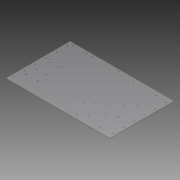
# Autodesk Inventor part: Mounting Board 1
Saved by Autodesk Inventor 2013 (Build 170138000, 138)
## iProperties
Created: 2013-01-21
Part Number: Mounting Board 1
Material: Polycarbonate, Clear
Document SubType Name: Modeling
Designer: Moses
Density: 1.2 g/cm^3
Mass: 570.089 g
Surface Area: 3065.39 cm^2
Volume: 475.074 cm^3
Author: Moses
Autodesk Inventor part; units mm, degrees
ref_plane "YZ Plane" through (0, 0, 0) normal (1, 0, 0) x (0, 1, 0)
ref_plane "XZ Plane" through (0, 0, 0) normal (0, 1, 0) x (-1, 0, 0)
ref_plane "XY Plane" through (0, 0, 0) normal (0, 0, 1) x (1, 0, 0)
sketch "Sketch1" plane through (0, 0, 0) normal (0, 1, 0) x (-1, 0, 0)
  line L0 (0, 0) -> (493.7125, 0)
  line L1 (493.7125, 0) -> (493.7125, 304.8)
  line L2 (0, 304.8) -> (0, 0)
  line L3 (0, 304.8) -> (493.7125, 304.8)
  circle A0 centre (42.8625, 261.9375) radius 1.905
  circle A1 centre (104.9909, 220.1291) radius 1.905
  line L4 (38.1, 266.7) -> (109.7534, 266.7) construction
  line L5 (109.7534, 266.7) -> (109.7534, 215.3666) construction
  line L6 (109.7534, 215.3666) -> (38.1, 215.3666) construction
  line L7 (38.1, 215.3666) -> (38.1, 266.7) construction
  circle A2 centre (252.4125, 219.075) radius 2.54
  circle A3 centre (379.4125, 219.075) radius 2.54
  circle A4 centre (252.4125, 9.525) radius 2.54
  circle A5 centre (379.4125, 9.525) radius 2.54
  line L8 (252.4125, 219.075) -> (379.4125, 219.075) construction
  line L9 (379.4125, 219.075) -> (379.4125, 9.525) construction
  line L10 (379.4125, 9.525) -> (252.4125, 9.525) construction
  line L11 (252.4125, 219.075) -> (252.4125, 9.525) construction
  circle A6 centre (144.4625, 261.9375) radius 1.905
  circle A7 centre (206.5909, 220.1291) radius 1.905
  line L12 (139.7, 266.7) -> (211.3534, 266.7) construction
  line L13 (211.3534, 266.7) -> (211.3534, 215.3666) construction
  line L14 (211.3534, 215.3666) -> (139.7, 215.3666) construction
  line L15 (139.7, 215.3666) -> (139.7, 266.7) construction
  circle A8 centre (42.8625, 173.0375) radius 1.905
  circle A9 centre (104.9909, 131.2291) radius 1.905
  line L16 (38.1, 177.8) -> (109.7534, 177.8) construction
  line L17 (109.7534, 177.8) -> (109.7534, 126.4666) construction
  line L18 (109.7534, 126.4666) -> (38.1, 126.4666) construction
  line L19 (38.1, 126.4666) -> (38.1, 177.8) construction
  circle A10 centre (144.4625, 173.0375) radius 1.905
  circle A11 centre (206.5909, 131.2291) radius 1.905
  line L20 (139.7, 177.8) -> (211.3534, 177.8) construction
  line L21 (211.3534, 177.8) -> (211.3534, 126.4666) construction
  line L22 (211.3534, 126.4666) -> (139.7, 126.4666) construction
  line L23 (139.7, 126.4666) -> (139.7, 177.8) construction
  circle A12 centre (42.8625, 84.1375) radius 1.905
  circle A13 centre (104.9909, 42.3291) radius 1.905
  line L24 (38.1, 88.9) -> (109.7534, 88.9) construction
  line L25 (109.7534, 88.9) -> (109.7534, 37.5666) construction
  line L26 (109.7534, 37.5666) -> (38.1, 37.5666) construction
  line L27 (38.1, 37.5666) -> (38.1, 88.9) construction
  circle A14 centre (144.4625, 84.1375) radius 1.905
  circle A15 centre (206.5909, 42.3291) radius 1.905
  line L28 (139.7, 88.9) -> (211.3534, 88.9) construction
  line L29 (211.3534, 88.9) -> (211.3534, 37.5666) construction
  line L30 (211.3534, 37.5666) -> (139.7, 37.5666) construction
  line L31 (139.7, 37.5666) -> (139.7, 88.9) construction
  line L32 (481.0125, 304.8) -> (481.0125, 0) construction
  circle A16 centre (481.0125, 279.4) radius 2.54
  line L33 (12.7, 304.8) -> (12.7, 0) construction
  circle A17 centre (12.7, 279.4) radius 2.54
  circle A18 centre (481.0125, 228.6) radius 2.54
  circle A19 centre (12.7, 228.6) radius 2.54
  circle A20 centre (481.0125, 177.8) radius 2.54
  circle A21 centre (12.7, 177.8) radius 2.54
  circle A22 centre (481.0125, 127) radius 2.54
  circle A23 centre (12.7, 127) radius 2.54
  line L34 (66.675, 285.4833) -> (66.675, 196.5833) construction
  circle A24 centre (66.675, 285.4833) radius 2.54
  circle A25 centre (66.675, 196.5833) radius 2.54
  line L35 (38.1, 241.0333) -> (109.7534, 241.0333) construction
  circle A26 centre (174.625, 285.4833) radius 2.54
  circle A27 centre (174.625, 196.5833) radius 2.54
  circle A28 centre (66.675, 107.6833) radius 2.54
  circle A29 centre (66.675, 18.7833) radius 2.54
  circle A30 centre (174.625, 107.6833) radius 2.54
  circle A31 centre (174.625, 18.7833) radius 2.54
  line L36 (406.0013, 241.3) -> (461.9625, 241.3) construction
  circle A32 centre (406.0013, 241.3) radius 3.302
  circle A33 centre (461.9625, 241.3) radius 3.302
  circle A34 centre (455.6125, 136.017) radius 2.54
  circle A35 centre (455.6125, 194.183) radius 2.54
  circle A36 centre (411.1625, 136.017) radius 2.54
  circle A37 centre (411.1625, 194.183) radius 2.54
  line L37 (455.6125, 136.017) -> (455.6125, 194.183) construction
  line L38 (411.1625, 136.017) -> (411.1625, 194.183) construction
  line L39 (411.1625, 165.1) -> (455.6125, 165.1) construction
  circle A38 centre (404.8125, 123.825) radius 2.54
  circle A39 centre (468.3125, 123.825) radius 2.54
  circle A40 centre (404.8125, 9.525) radius 2.54
  circle A41 centre (468.3125, 9.525) radius 2.54
  circle A42 centre (481.0125, 76.2) radius 2.54
  circle A43 centre (12.7, 76.2) radius 2.54
  circle A44 centre (481.0125, 25.4) radius 2.54
  circle A45 centre (12.7, 25.4) radius 2.54
  point P0 (66.675, 241.0333)
  dimension "d0" = 304.8
  dimension "d4" = 493.7125
  dimension "d6" = 3.81
  dimension "d7" = 3.81
  dimension "d8" = 41.8084
  dimension "d9" = 62.1284
  dimension "d11" = 4.7625
  dimension "d12" = 4.7625
  dimension "d13" = 4.7625
  dimension "d14" = 4.7625
  dimension "d15" = 38.1
  dimension "d16" = 38.1
  dimension "d17" = 209.55
  dimension "d18" = 127
  dimension "d19" = 5.08
  dimension "d20" = 114.3
  dimension "d21" = 9.525
  dimension "d24" = 101.6
  dimension "d27" = 88.9
  dimension "d32" = 12.7
  dimension "d33" = 5.08
  dimension "d34" = 25.4
  dimension "d35" = 12.7
  dimension "d37" = 25.4
  dimension "d43" = 50.8
  dimension "d45" = 88.9
  dimension "d46" = 5.08
  dimension "d49" = 107.95
  dimension "d52" = 177.8
  dimension "d55" = 18.7833
  dimension "d56" = 18.7833
  dimension "d57" = 55.9612
  dimension "d58" = 6.604
  dimension "d59" = 241.3
  dimension "d63" = 5.08
  dimension "d67" = 165.1
  dimension "d68" = 31.75
  dimension "d69" = 58.166
  dimension "d70" = 44.45
  dimension "d71" = 25.4
  dimension "d72" = 53.975
  dimension "d75" = 63.5
  dimension "d78" = 114.3
  dimension "d81" = 5.08
  dimension "d82" = 123.825
  dimension "d83" = 25.4
  constraints: 80 end point, 46 centre point, 9 equal radius, 9 parallel, 7 horizontal, 7 point on line, 6 vertical, 5 midpoint, 5 perpendicular, 4 coincident, 98 other
  measures "d0" distance of L2.start L0.start
  measures "d4" distance of L0.start L0.end
  measures "d6" diameter of A0
  measures "d7" diameter of A1
  measures "d8" vertical distance of A1.centre A0.centre
  measures "d9" horizontal distance of A1.centre A0.centre
  measures "d11" distance from line of L4 A0.centre
  measures "d12" distance from line of A0.centre L7
  measures "d13" distance from line of L6 A1.centre
  measures "d14" distance from line of L5 A1.centre
  measures "d15" distance between parallel lines of L3 L4
  measures "d16" distance between parallel lines of L7 L2
  measures "d17" distance of L10.end L8.start
  measures "d18" distance of L8.start L8.end
  measures "d19" diameter of A2
  measures "d20" distance between parallel lines of L1 L9
  measures "d21" distance between parallel lines of L0 L10
  measures "d24" distance of L4.end L13.start
  measures "d27" distance of L4.end L17.start
  measures "d32" distance between parallel lines of L1 L32
  measures "d33" diameter of A16
  measures "d34" distance from line of A16.centre L3
  measures "d35" distance between parallel lines of L33 L2
  measures "d37" distance from line of L3 A17.centre
  measures "d43" distance of A17.centre A19.centre
  measures "d45" distance of L34.start L34.end
  measures "d46" diameter of A24
  measures "d49" distance of A24.centre A26.centre
  measures "d52" distance of A24.centre A28.centre
  measures "d55" distance from line of L24 A28.centre
  measures "d56" distance from line of L26 A29.centre
  measures "d57" distance of L36.start L36.end
  measures "d58" diameter of A32
  measures "d59" distance between parallel lines of L0 L36
  measures "d63" diameter of A34
  measures "d67" distance between parallel lines of L0 L39
  measures "d68" distance from line of L1 L36.end
  measures "d69" distance of L38.start L38.end
  measures "d70" distance of L39.start L39.end
  measures "d71" distance between parallel lines of L32 L37
  measures "d72" distance between parallel lines of L34 L33
  measures "d75" distance of A38.centre A39.centre
  measures "d78" distance of A38.centre A40.centre
  measures "d81" diameter of A38
  measures "d82" distance from line of L0 A38.centre
  measures "d83" distance from line of L1 A39.centre
extrude "Extrusion1" add sketch "Sketch1" along normal blind 3.175
equation "\"d7\" = d6"
equation "\"d11\" = d12"
equation "\"d13\" = d12"
equation "\"d14\" = d12"
equation "\"d37\" = d34"
body "Solid1"
